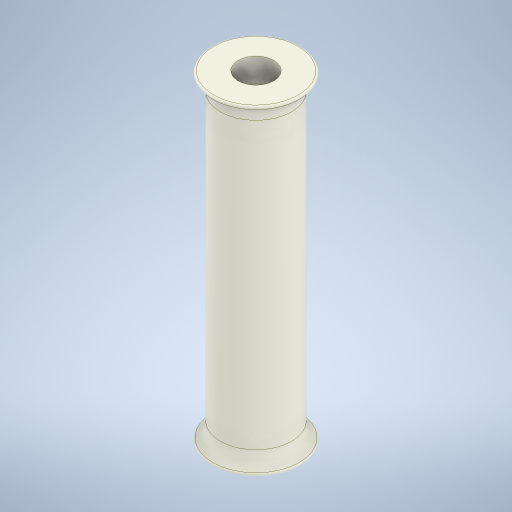
# Autodesk Inventor part: Top Level Pegs
Saved by Autodesk Inventor 2024 (Build 280153000, 153)
## iProperties
Created: 2023-08-02
Part Number: Top Level Pegs
Material: PET Plastic
Document SubType Name: Modeling
Designer: javie
Density: 1.541 g/cm^3
Appearance: Smooth - Ivory
Author: javie
Autodesk Inventor part; units mm, degrees
ref_plane "YZ Plane" through (0, 0, 0) normal (1, 0, 0) x (0, 1, 0)
ref_plane "XZ Plane" through (0, 0, 0) normal (0, 1, 0) x (-1, 0, 0)
ref_plane "XY Plane" through (0, 0, 0) normal (0, 0, 1) x (1, 0, 0)
sketch "Sketch1" plane through (0, 0, 0) normal (0, 0, 1) x (1, 0, 0)
  line L0 (0, -20) -> (-5, -20)
  line L1 (-5, -20) -> (-5, 20)
  line L2 (-5, 20) -> (0, 20)
  line L3 (0, 20) -> (0, -20)
  circle A0 centre (-2.5, 20) radius 2.5
  line L4 (-5.9189, 22.5) -> (0, 22.5)
  arc A1 (-5, 20) -> (-6.0626, 22.0455) centre (-7.5, 20) ccw
  arc A2 (-5.9189, 22.5) -> (-6.0626, 22.0455) centre (-5.9189, 22.25) ccw
  line L5 (0, 20) -> (0, 22.5)
  circle A3 centre (-2.5, -20) radius 2.5
  line L6 (-5.9189, -22.5) -> (0, -22.5)
  line L7 (0, -22.5) -> (0, -20)
  arc A4 (-6.0626, -22.0455) -> (-5, -20) centre (-7.5, -20) ccw
  arc A5 (-6.0626, -22.0455) -> (-5.9189, -22.5) centre (-5.9189, -22.25) ccw
  point P0 (0, 0)
  point P1 (0, 0)
  point P2 (-7.5, 22.5)
  point P3 (-7.5, -22.5)
  dimension "d0" = 5
  dimension "d1" = 40
  dimension "d2" = 5
  dimension "d3" = 7.5
  dimension "d4" = 0.25
  dimension "d5" = 2.5
  dimension "d6" = 5
  dimension "d7" = 7.5
  dimension "d8" = 0.25
  constraints: 16 end point, 10 point on circle, 9 tangent, 6 centre point, 3 horizontal, 3 midpoint, 2 parallel, 2 point on line, 1 coincident, 1 perpendicular
  measures "d0" distance of L1.end L2.end
  measures "d1" distance of L0.end L1.end
  measures "d2" diameter of A0
  measures "d3" distance of L4.end point (-7.5, 22.5)
  measures "d4" radius of A2
  measures "d5" distance of L2.end L4.end
  measures "d6" diameter of A3
  measures "d7" distance of point (-7.5, -22.5) L6.end
  measures "d8" radius of A5
revolve "Revolution1" add sketch "Sketch1" angle 360 about axis through (0, 20, 0) along (0, -1, 0)
sketch "Sketch2" plane through (0, 22.5, 0) normal (0, 1, 0) x (1, 0, 0)
  point P0 (0, 0)
  point P1 (0, 0)
  constraints: 1 coincident
hole "Hole1" at (0, 22.5, 0) direction (0, -1, 0) diameter 5 end through all
equation "\"d0\" = Scaler"
equation "\"d2\" = Scaler"
equation "\"d3\" = 15 * Scaler"
equation "\"d4\" = 0.5 * Scaler"
equation "\"d5\" = 5 * Scaler"
equation "\"d6\" = Scaler"
equation "\"d7\" = 15 * Scaler"
equation "\"d8\" = 0.5 * Scaler"
equation "\"Scaler\" = 0.5"
